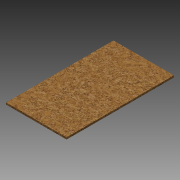
# Autodesk Inventor part: srodek
Saved by Autodesk Inventor 2013 (Build 170138000, 138)
## iProperties
Created: 2014-04-26
Part Number: srodek
Material: Generic
Document SubType Name: Modeling
Designer: Masta
Density: 1 g/cm^3
Author: Masta
Autodesk Inventor part; units mm, degrees
ref_plane "YZ Plane" through (0, 0, 0) normal (1, 0, 0) x (0, 1, 0)
ref_plane "XZ Plane" through (0, 0, 0) normal (0, 1, 0) x (-1, 0, 0)
ref_plane "XY Plane" through (0, 0, 0) normal (0, 0, 1) x (1, 0, 0)
sketch "Sketch1" plane through (0, 0, 0) normal (0, 0, 1) x (1, 0, 0)
  line L0 (-282, -501) -> (282, -501)
  line L1 (282, -501) -> (282, 501)
  line L2 (282, 501) -> (-282, 501)
  line L3 (-282, 501) -> (-282, -501)
  line L4 (-282, -501) -> (282, 501) construction
  line L5 (282, -501) -> (-282, 501) construction
  point P0 (0, 0)
  dimension "d0" = 564
  dimension "d1" = 1002
  constraints: 12 end point, 2 midpoint, 2 parallel, 1 horizontal, 1 perpendicular
  measures "d0" distance of L2.end L1.end
  measures "d1" distance of L1.end L0.end
extrude "Extrusion1" add sketch "Sketch1" along normal blind 18
body "Solid1"
